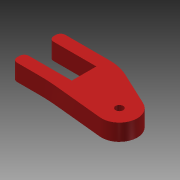
# Autodesk Inventor part: Soportes filamento
Saved by Autodesk Inventor 2014 (Build 180170000, 170)
## iProperties
Created: 2014-09-27
Part Number: Soportes filamento
Material: Generic
Document SubType Name: Modeling
Designer: Rubén
Density: 1 g/cm^3
Appearance: Light Red
Author: Rubén
Autodesk Inventor part; units mm, degrees
ref_plane "YZ Plane" through (0, 0, 0) normal (1, 0, 0) x (0, 1, 0)
ref_plane "XZ Plane" through (0, 0, 0) normal (0, 1, 0) x (-1, 0, 0)
ref_plane "XY Plane" through (0, 0, 0) normal (0, 0, 1) x (1, 0, 0)
sketch "Sketch10" plane through (0, 0, 0) normal (0, 1, 0) x (-1, 0, 0)
  circle A0 centre (0, 0) radius 1.6
  arc A1 (0.7577, 7.4616) -> (-3.1789, -6.793) centre (0, 0) ccw
  line L0 (0, 0) -> (0, -7.5) construction
  line L1 (0, 0) -> (7.5, 0) construction
  line L2 (0, 0) -> (63.5588, 0) construction
  line L3 (40, 0) -> (20, 0)
  line L4 (20, 0) -> (20, -10.3)
  line L5 (20, -10.3) -> (40, -10.3)
  line L6 (40, -10.3) -> (40, -15.3)
  line L7 (40, -15.3) -> (19.4481, -15.3)
  line L8 (10.9712, -13.4147) -> (-3.1789, -6.793)
  line L9 (40, 0) -> (40, 5)
  line L10 (40, 5) -> (29.0513, 5)
  line L11 (20.9694, 5.4093) -> (0.7577, 7.4616)
  arc A2 (20.9694, 5.4093) -> (29.0513, 5) centre (29.0513, 85) ccw
  arc A3 (10.9712, -13.4147) -> (19.4481, -15.3) centre (19.4481, 4.7) ccw
  point P0 (15, -15.3)
  point P1 (25, 5)
  dimension "d117" = 3.2
  dimension "d118" = 15
  dimension "d120" = 10.3
  dimension "d121" = 20
  dimension "d122" = 0
  dimension "d123" = 20
  dimension "d124" = 5
  dimension "d125" = 5
  dimension "d126" = 25
  dimension "d127" = 15
  dimension "d128" = 80
  dimension "d129" = 20
  dimension "d133" = 0
  constraints: 24 end point, 7 point on line, 6 point on circle, 6 tangent, 4 centre point, 3 parallel, 3 vertical, 2 coincident, 2 perpendicular, 1 collinear
  measures "d117" diameter of A0
  measures "d118" diameter of A1
  measures "d120" distance of L3.end L4.end
  measures "d121" distance from line of point (0, 0) L4
  measures "d122" horizontal distance of L5.end L3.start
  measures "d123" distance of L3.start L3.end
  measures "d124" distance of L3.start L9.end
  measures "d125" distance of L5.end L6.end
  measures "d126" distance of L6.end point (15, -15.3)
  measures "d127" distance of L9.end point (25, 5)
  measures "d128" radius of A2
  measures "d129" radius of A3
  measures "d133" distance between parallel lines of L1 L2
extrude "Extrusion7" add sketch "Sketch10" along normal blind 7
fillet "Fillet5" radius 2 4 edges at (-40, 3.5, 5) (-40, 3.5, 0) (-40, 3.5, -10.3) (-40, 3.5, -15.3)
body "Solid2"
